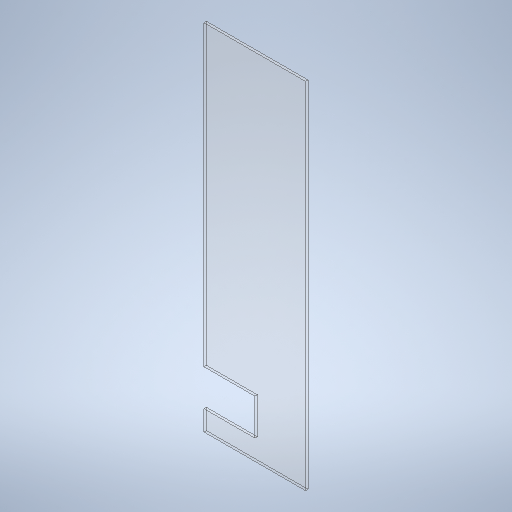
# Autodesk Inventor part: ackleryk
Saved by Autodesk Inventor 2025.4 (Build 294407000, 407)
## iProperties
Created: 2026-04-12
Part Number: ackleryk
Material: PMMA Plastic
Document SubType Name: Modeling
Designer: abdo2
Density: 1.188 g/cm^3
Appearance: Polycarbonate - Clear
Author: abdo2
Autodesk Inventor part; units mm, degrees
ref_plane "YZ Plane" through (0, 0, 0) normal (1, 0, 0) x (0, 1, 0)
ref_plane "XZ Plane" through (0, 0, 0) normal (0, 1, 0) x (-1, 0, 0)
ref_plane "XY Plane" through (0, 0, 0) normal (0, 0, 1) x (1, 0, 0)
sketch "Sketch2" plane through (0, 0, 0) normal (0, 0, 1) x (1, 0, 0)
  line L0 (0, 0) -> (126, 0)
  line L1 (126, 0) -> (126, 439)
  line L2 (126, 439) -> (0, 439)
  line L3 (0, 439) -> (0, 0)
  line L4 (0, 25) -> (63, 25)
  line L5 (63, 0) -> (0, 0)
  line L6 (0, 0) -> (0, 25)
  line L7 (63, 25) -> (63, 70)
  line L8 (63, 70) -> (0, 70)
  point P0 (63, 47.5)
  dimension "d0" = 126
  dimension "d1" = 439
  dimension "d2" = 25
  dimension "d3" = 45
  dimension "d4" = 63
  constraints: 18 end point, 3 parallel, 2 horizontal, 2 midpoint, 2 perpendicular, 2 point on line, 1 vertical
  measures "d0" distance of L2.end L1.end
  measures "d1" distance of L1.end L0.end
  measures "d2" distance between parallel lines of L0 L4
  measures "d3" distance of L4.end L7.end
  measures "d4" distance from line of L1 point (63, 47.5)
extrude "Extrusion1" add sketch "Sketch2" along normal blind 3 contours L3 L4 L7 L8 L2 L1 L0
body "Solid1"
